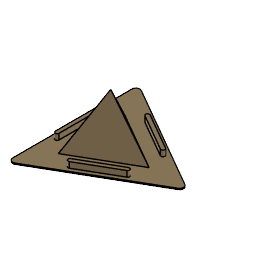
Phone Stand (Autodesk Fusion 360 design; units mm, degrees)
part number: 2026-06-28-14-59-09-436
Autodesk Fusion 360 part; units mm, degrees
sketch "Sketch1" plane through (0, 0, 0) normal (0, 0, 1) x (1, 0, 0)
  line L0 (200, 0) -> (-100, 173.2051)
  line L1 (-100, 173.2051) -> (-100, -173.2051)
  line L2 (-100, -173.2051) -> (200, 0)
  dimension "d15" = 200
  measures "d15" distance of L0.start origin
extrude "Extrude1" add sketch "Sketch1" along normal blind 3
sketch "Sketch2" plane through (0, 0, 3) normal (0, 0, 1) x (-1, 0, 0)
  line L0 (100, 173.2051) -> (-200, 0)
  line L1 (-200, 0) -> (100, -173.2051)
  line L2 (100, -173.2051) -> (100, 173.2051)
  line L3 (-75, 0) -> (37.5, -64.9519)
  line L4 (37.5, -64.9519) -> (37.5, 64.9519)
  line L5 (37.5, 64.9519) -> (-75, 0)
sketch "Sketch3" plane through (0, 0, 0) normal (0, 1, 0) x (1, 0, 0)
sketch "Sketch4" plane through (0, 0, 3) normal (0, 0, 1) x (-1, 0, 0)
sketch "Sketch5" plane through (0, 0, 3) normal (0, 0, 1) x (1, 0, 0)
sketch "Sketch6" plane through (0, 0, 0) normal (0, 1, 0) x (1, 0, 0)
  line L0 (0, 0) -> (0, -100)
  dimension "d19" = 100
  constraint coincident L0.start origin
  constraint vertical L0
  measures "d19" distance of L0.start L0.end
loft "Loft1" add profiles "Sketch2" section 1 contours L3 L4 L5 section 2 point at (0, 0, 100)
delete_face "DeleteFace1" 1 faces at (-25, 0, 35.3333)
sketch "Sketch7" plane through (0, 0, 3) normal (0, 0, 1) x (-1, 0, 0)
  line L0 (100, 173.2051) -> (-200, 0)
  line L1 (-200, 0) -> (100, -173.2051)
  line L2 (100, -173.2051) -> (100, 173.2051)
  line L3 (-100, 0) -> (50, -86.6025)
  line L4 (50, -86.6025) -> (50, 86.6025)
  line L5 (50, 86.6025) -> (-100, 0)
sketch "Sketch8" plane through (0, 0, 0) normal (0, 1, 0) x (1, 0, 0)
  line L0 (0, 0) -> (0, -130)
  dimension "d20" = 130
  constraint coincident L0.start origin
  constraint vertical L0
  measures "d20" distance of L0.start L0.end
loft "Loft2" add profiles "Sketch7" section 1 contours L3 L4 L5 section 2 point at (0, 0, 130)
sketch "Sketch9" plane through (0, 0, 3) normal (0, 0, 1) x (-1, 0, 0)
  line L0 (-100, 0) -> (50, 86.6025)
  line L1 (50, 86.6025) -> (50, -86.6025)
  line L2 (50, -86.6025) -> (-100, 0)
  line L3 (100, 173.2051) -> (-200, 0)
  line L4 (-200, 0) -> (100, -173.2051)
  line L5 (100, -173.2051) -> (100, 173.2051)
  line L6 (90, 60) -> (90, -60)
  line L7 (90, -60) -> (80, -60)
  line L8 (80, -60) -> (80, 60)
  line L9 (80, 60) -> (90, 60)
  line L10 (6.9615, 107.9423) -> (-96.9615, 47.9423)
  line L11 (-96.9615, 47.9423) -> (-91.9615, 39.282)
  line L12 (6.9615, 107.9423) -> (11.9615, 99.282)
  line L13 (11.9615, 99.282) -> (-91.9615, 39.282)
  line L14 (6.9615, -107.9423) -> (-96.9615, -47.9423)
  line L15 (6.9615, -107.9423) -> (11.9615, -99.282)
  line L16 (-96.9615, -47.9423) -> (-91.9615, -39.282)
  line L17 (11.9615, -99.282) -> (-91.9615, -39.282)
  constraint perpendicular L6 L7
  constraint perpendicular L7 L8
  constraint perpendicular L6 L9
  constraint perpendicular L10 L11
  constraint perpendicular L10 L12
  constraint perpendicular L14 L15
  constraint perpendicular L14 L16
extrude "Extrude2" add sketch "Sketch9" along normal blind 15 contours L6 L7 L8 L9 | L10 L11 L12 L13 | L14 L15 L16 L17
fillet "Fillet1" radius 10 3 edges at (-100, -173.2051, 1.5) (-100, 173.2051, 1.5) (200, 0, 1.5)
fillet "Fillet2" radius 5 12 edges at (-6.9615, 107.9423, 10.5) (-11.9615, 99.282, 10.5) (-80, 60, 10.5) (-90, 60, 10.5) (-90, -60, 10.5) (-80, -60, 10.5) (-11.9615, -99.282, 10.5) (-6.9615, -107.9423, 10.5) (96.9615, -47.9423, 10.5) (91.9615, -39.282, 10.5) (91.9615, 39.282, 10.5) (96.9615, 47.9423, 10.5)
